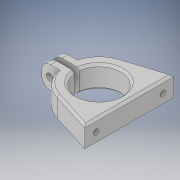
# Autodesk Inventor part: BasicMount 40mm
Saved by Autodesk Inventor 2019.3 (Build 233278000, 278)
## iProperties
Created: 2019-04-04
Part Number: BasicMount 40mm
Material: Типовые
Document SubType Name: Modeling
Designer: Andrew
Density: 1 g/cm^3
Appearance: По умолчанию
Author: Andrew
## iProperties of the stored document BasicMount 40mm_3DПЕЧАТЬ.ipt
Created: 2019-04-16
Part Number: BasicMount 40mm_3DПЕЧАТЬ
Material: Типовые
Document SubType Name: Modeling
Designer: Andrew
Density: 1 g/cm^3
Appearance: По умолчанию
Author: Andrew
Autodesk Inventor part; units mm, degrees
ref_plane "YZ Plane" through (0, 0, 0) normal (1, 0, 0) x (0, 1, 0)
ref_plane "XZ Plane" through (0, 0, 0) normal (0, 1, 0) x (-1, 0, 0)
ref_plane "XY Plane" through (0, 0, 0) normal (0, 0, 1) x (1, 0, 0)
sketch "Эскиз1" plane through (0, 0, 0) normal (0, 1, 0) x (-1, 0, 0)
  arc A0 (9.8249, 1.217) -> (9.8505, -0.9889) centre (0, 0) ccw
  line L0 (-13.6311, 20) -> (-13.6311, -20)
  line L1 (-13.6311, 20) -> (4.492, 14.3116)
  line L2 (-13.6311, -20) -> (4.492, -14.3116)
  line L3 (9.8249, 1.217) -> (16.2051, 1.217)
  line L4 (13.6718, -0.9889) -> (9.8505, -0.9889)
  arc A1 (4.492, -14.3116) -> (14.5136, -3.7889) centre (0, 0) ccw
  arc A2 (14.4521, 4.017) -> (4.492, 14.3116) centre (0, 0) ccw
  line L5 (9.8505, -0.9889) -> (21.6521, -0.9889)
  line L6 (21.6521, -0.9889) -> (21.6521, -3.7889)
  line L7 (21.6521, -3.7889) -> (14.5136, -3.7889)
  line L8 (9.8249, 1.217) -> (21.6265, 1.217)
  line L9 (21.6265, 1.217) -> (21.6265, 4.017)
  line L10 (21.6265, 4.017) -> (14.4521, 4.017)
  point P0 (15, 0)
  dimension "d0" = 19.8
  dimension "d5" = 2.8
  dimension "d6" = 2.8
  dimension "d32" = 15
  dimension "d33" = 40
  constraints: 22 end point, 6 point on circle, 3 centre point, 3 horizontal, 3 parallel, 2 coincident, 2 equal length, 2 perpendicular, 2 tangent, 1 concentric, 1 vertical
  measures "d0" diameter of A0
  measures "d5" distance between parallel lines of L7 L5
  measures "d6" distance of L8.end L9.end
  measures "d32" radius of A1
  measures "d33" distance of L0.start L0.end
extrude "Выдавливание1" add sketch "Эскиз1" along normal blind 10
fillet "Сопряжение1" radius 4 4 edges at (-21.6265, 10, 2.617) (-21.6521, 10, -2.3889) (-21.6265, 0, 2.617) (-21.6521, 0, -2.3889)
sketch "Эскиз3" plane through (-14.4521, 0, 4.017) normal (0, 0, 1) x (1, 0, 0)
  arc A0 (-7.1744, 4) -> (-3.1744, 0) centre (-3.1744, 4) ccw projected
  line L0 (-3.1744, 0) -> (0, 0) projected
  line L1 (0, 0) -> (0, 10) projected
  line L2 (-3.1744, 10) -> (0, 10) projected
  arc A1 (-3.1744, 10) -> (-7.1744, 6) centre (-3.1744, 6) ccw projected
  line L3 (-7.1744, 4) -> (-7.1744, 6) projected
  line L4 (-7.1744, 5) -> (-3.6744, 5) construction
  point P0 (14.4521, 0)
  dimension "d20" = 3.5
  constraints: 2 end point, 1 coincident, 1 horizontal, 1 midpoint
  measures "d20" distance of L4.start L4.end
hole "Отверстие2" at (-18.1265, 5, 4.017) direction (0, 0, -1) diameter 3 depth 8 tip angle 118
chamfer "Фаска1" distance 1 angle 45 12 edges at (9.8993, 10, -0.1148) (9.8993, 0, -0.1148) (4.5696, 10, 17.1558) (13.6311, 10, 0) (4.5696, 10, -17.1558) (-10.8621, 10, -10.3448) (-10.7803, 10, 10.43) (4.5696, 0, 17.1558) (13.6311, 0, 0) (4.5696, 0, -17.1558) (-10.8621, 0, -10.3448) (-10.7803, 0, 10.43)
sketch "Эскиз5" plane through (13.6311, 1, -20) normal (1, 0, 0) x (0, 0, -1)
  line L0 (0, 0) -> (-40, 0) projected
  line L1 (0, 0) -> (0, 8) projected
  line L2 (-40, 8) -> (0, 8) projected
  line L3 (-40, 0) -> (-40, 8) projected
  line L4 (-35, 4) -> (-40, 4) construction
  line L5 (-5, 4) -> (0, 4) construction
  line L6 (-5, 8) -> (-5, 4) construction
  line L7 (-5, 4) -> (-5, 0) construction
  point P0 (-20, -1)
  dimension "d34" = 30
  constraints: 8 end point, 3 point on line, 2 collinear, 2 midpoint, 2 perpendicular, 1 horizontal
  measures "d34" distance of L5.start L4.start
hole "Отверстие3" at (13.6311, 5, 15) at (13.6311, 5, -15) direction (-1, 0, 0) diameter 2.4 depth 8 tip angle 118
